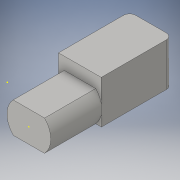
# Autodesk Inventor part: cwmotor
Saved by Autodesk Inventor 2016 (Build 200138000, 138)
## iProperties
Created: 2017-09-05
Part Number: cwmotor
Material: Generic
Document SubType Name: Modeling
Designer: student
Density: 1 g/cm^3
Appearance: Default
Author: student
Autodesk Inventor part; units mm, degrees
ref_plane "YZ Plane" through (0, 0, 0) normal (1, 0, 0) x (0, 1, 0)
ref_plane "XZ Plane" through (0, 0, 0) normal (0, 1, 0) x (-1, 0, 0)
ref_plane "XY Plane" through (0, 0, 0) normal (0, 0, 1) x (1, 0, 0)
sketch "Sketch1" plane through (0, 0, 0) normal (0, 0, 1) x (1, 0, 0)
  line L0 (-8.128, 7.8935) -> (8.128, 7.8935)
  line L1 (-8.0668, -7.9561) -> (8.0668, -7.9561)
  arc A0 (-8.128, 7.8935) -> (-8.0668, -7.9561) centre (0, 0) ccw
  arc A1 (8.0668, -7.9561) -> (8.128, 7.8935) centre (0, 0) ccw
  line L2 (0, 7.8935) -> (0, -7.9561)
  dimension "d8" = 15.8496
  dimension "d9" = 16.256
  constraints: 6 end point, 4 point on circle, 2 centre point, 2 horizontal, 2 midpoint, 1 coincident
  measures "d8" distance of L2.start L2.end
  measures "d9" distance of L0.start L0.end
extrude "Extrusion1" add sketch "Sketch1" along normal blind 26.4922
sketch "Sketch2" plane through (0, 0, 0) normal (0, 0, -1) x (-0.0038611, 0.9999925, 0)
  line L0 (-7.956, -11.1178) -> (14.2944, -11.1178)
  line L1 (14.2944, -11.1178) -> (14.2944, 11.0564)
  line L2 (14.2944, 11.0564) -> (-7.956, 11.0564)
  line L3 (-7.956, 11.0564) -> (-7.956, -11.1178)
  line L4 (-4.7868, -0.0614) -> (-7.956, -0.0307)
  point P0 (0, 0)
  dimension "d3" = 22.2504
  dimension "d4" = 22.1742
  constraints: 10 end point, 2 parallel, 1 horizontal, 1 midpoint, 1 perpendicular
  measures "d3" distance of L1.end L2.end
  measures "d4" distance of L0.end L1.end
extrude "Extrusion2" add sketch "Sketch2" along normal blind 36.83
fillet "Fillet1" radius 3.175 2 edges at (-11.13, 3.1262, -36.83) (11.0441, 3.2119, -36.83)
sketch "Sketch4" plane through (0, 0, 26.4922) normal (0, 0, 1) x (0.0038611, -0.9999925, 0)
  point P0 (0, 0)
  point P1 (-14.2944, -11.1178)
sketch "Sketch6" plane through (11.087, -7.9133, -33.655) normal (0.0038611, -0.9999925, 0) x (0.9999925, 0.0038611, 0)
  line L0 (-13.3136, 11.6068) -> (-8.7992, 11.6068)
  line L1 (-13.8088, 7.0188) -> (-8.3039, 7.0188)
  arc A0 (-13.3136, 11.6068) -> (-13.8088, 7.0188) centre (-11.0564, 9.0424) ccw
  arc A1 (-8.3039, 7.0188) -> (-8.7992, 11.6068) centre (-11.0564, 9.0424) ccw
  point P0 (-11.0564, 33.655)
  constraints: 4 end point, 4 point on circle, 2 centre point, 2 horizontal
extrude "Extrusion3" add sketch "Sketch6" along normal blind 5.207
body "Solid1"
